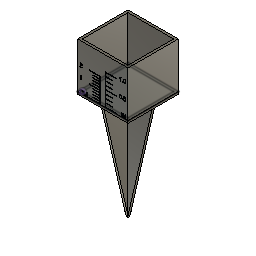
SprinklerGage (Autodesk Fusion 360 design; units mm, degrees)
Autodesk Fusion 360 part; units mm, degrees
sketch "Sketch1" plane through (0, 0, 0) normal (0, 0, 1) x (1, 0, 0)
  line L0 (0, 0) -> (38.1, 0)
  line L1 (38.1, 0) -> (38.1, 38.1)
  line L2 (38.1, 38.1) -> (0, 38.1)
  line L3 (0, 38.1) -> (0, 0)
  line L4 (-2, -2) -> (40.1, -2)
  line L5 (40.1, -2) -> (40.1, 40.1)
  line L6 (40.1, 40.1) -> (-2, 40.1)
  line L7 (-2, 40.1) -> (-2, -2)
  dimension "d6" = 38.1
  dimension "d7" = 38.1
  dimension "d8" = 2
  constraint horizontal L0
  constraint vertical L1
  constraint horizontal L2
  constraint vertical L3
  constraint coincident L0.start L3.end
  measures "d6" distance of L0.start L0.end
  measures "d7" distance of L0.start L2.end
extrude "Extrude1" add sketch "Sketch1" along normal blind 38.1 makes body 1
extrude "Extrude2" add sketch "Sketch1" against normal blind 2 contours L0 L1 L2 L3 | L4 L5 L6 L7 bodies 1
sketch "Sketch2" plane through (0, 0, -2) normal (0, 0, -1) x (1, 0, 0)
  line L0 (-2, 2) -> (-2, -40.1)
  line L1 (-2, -40.1) -> (40.1, -40.1)
  line L2 (40.1, -40.1) -> (40.1, 2)
  line L3 (40.1, 2) -> (-2, 2)
  line L4 (-2, 2) -> (18.05, 2)
  line L5 (18.05, 2) -> (18.05, -18.05)
  line L6 (18.05, -18.05) -> (-2, -18.05)
  line L7 (-2, -18.05) -> (-2, 2)
  line L8 (-2, -40.1) -> (18.05, -40.1)
  line L9 (18.05, -40.1) -> (18.05, -20.05)
  line L10 (18.05, -20.05) -> (-2, -20.05)
  line L11 (-2, -20.05) -> (-2, -40.1)
  line L12 (40.1, -40.1) -> (20.05, -40.1)
  line L13 (20.05, -40.1) -> (20.05, -20.05)
  line L14 (20.05, -20.05) -> (40.1, -20.05)
  line L15 (40.1, -20.05) -> (40.1, -40.1)
  line L16 (40.1, 2) -> (20.05, 2)
  line L17 (20.05, 2) -> (20.05, -18.05)
  line L18 (20.05, -18.05) -> (40.1, -18.05)
  line L19 (40.1, -18.05) -> (40.1, 2)
  dimension "d14" = 20.05
  dimension "d15" = 20.05
  dimension "d16" = 20.05
  dimension "d17" = 20.05
  dimension "d18" = 20.05
  dimension "d19" = 20.05
  dimension "d20" = 20.05
  dimension "d21" = 20.05
  constraint horizontal L4
  constraint vertical L5
  constraint horizontal L6
  constraint vertical L7
  constraint coincident L0.start L3.end
  constraint horizontal L8
  constraint vertical L9
  constraint horizontal L10
  constraint vertical L11
  constraint coincident L0.end L1.start
  constraint horizontal L12
  constraint vertical L13
  constraint horizontal L14
  constraint vertical L15
  constraint coincident L1.end L2.start
  constraint horizontal L16
  constraint vertical L17
  constraint horizontal L18
  constraint vertical L19
  constraint coincident L2.end L3.start
  measures "d14" distance of L0.start L4.end
  measures "d15" distance of L0.start L6.end
  measures "d16" distance of L0.end L8.end
  measures "d17" distance of L0.end L10.end
  measures "d18" distance of L1.end L12.end
  measures "d19" distance of L1.end L14.end
  measures "d20" distance of L2.end L16.end
  measures "d21" distance of L2.end L18.end
extrude "Extrude3" add sketch "Sketch2" along normal blind 88.9 separate body contours L0 L1 L2 L3 L5 L6 L9 L10 L13 L14 L17 L18 makes body 2
draft "Draft1" angle 13 neutral plane through (0, 0, -2) pull (0, 0, -1) 4 faces at (-2, 18.7167, -31.6333) (18.7167, 40.1, -31.6333) (40.1, 19.3833, -31.6333) (19.3833, -2, -31.6333) on bodies 2
sketch "Sketch3" plane through (0, -2, 0) normal (0, -1, 0) x (1, 0, 0)
  line L0 (40.1, -2) -> (40.1, 38.1)
  line L1 (40.1, 38.1) -> (-2, 38.1)
  line L2 (-2, 38.1) -> (-2, -2)
  line L3 (-2, -2) -> (40.1, -2)
  line L4 (-2, 0) -> (40.1, 0)
  line L5 (21.05, 0) -> (21.05, 25.4)
  line L6 (21.55, 0) -> (21.55, 25.4)
  line L7 (21.05, 0) -> (30.575, 0)
  line L8 (30.575, 0) -> (30.575, 0.5)
  line L9 (30.575, 0.5) -> (21.05, 0.5)
  line L10 (21.05, 0.5) -> (21.05, 0)
  line L11 (21.05, 25.4) -> (30.575, 25.4)
  line L12 (30.575, 25.4) -> (30.575, 25.9)
  line L13 (30.575, 25.9) -> (21.05, 25.9)
  line L14 (21.05, 25.9) -> (21.05, 25.4)
  line L15 (17.05, 0) -> (17.05, 20)
  line L16 (16.55, 0) -> (16.55, 20)
  line L17 (17.05, 0) -> (7.525, 0)
  line L18 (7.525, 0) -> (7.525, 0.5)
  line L19 (7.525, 0.5) -> (17.05, 0.5)
  line L20 (17.05, 0.5) -> (17.05, 0)
  line L21 (17.05, 20) -> (7.525, 20)
  line L22 (7.525, 20) -> (7.525, 20.5)
  line L23 (7.525, 20.5) -> (17.05, 20.5)
  line L24 (17.05, 20.5) -> (17.05, 20)
  line L25 (35.4718, 0) -> (38.195, 0) construction
  line L26 (38.195, 0) -> (38.195, 1.9986) construction
  line L27 (38.195, 1.9986) -> (35.4718, 1.9986) construction
  line L28 (35.4718, 1.9986) -> (35.4718, 0) construction
  line L29 (-0.095, 0) -> (3.87, 0) construction
  line L30 (3.87, 0) -> (3.87, 2) construction
  line L31 (3.87, 2) -> (-0.095, 2) construction
  line L32 (-0.095, 2) -> (-0.095, 0) construction
  line L33 (32.2448, 25.3469) -> (38.2256, 25.3396) construction
  line L34 (38.2256, 25.3396) -> (38.2281, 27.4199) construction
  line L35 (38.2281, 27.4199) -> (32.2474, 27.4272) construction
  line L36 (32.2474, 27.4272) -> (32.2448, 25.3469) construction
  line L37 (-0.095, 19.9302) -> (2.7186, 20.0383) construction
  line L38 (2.7186, 20.0383) -> (2.6413, 22.0491) construction
  line L39 (2.6413, 22.0491) -> (-0.1722, 21.9411) construction
  line L40 (-0.1722, 21.9411) -> (-0.095, 19.9302) construction
  line L41 (17.05, 10) -> (7.525, 10)
  line L42 (7.525, 10) -> (7.525, 10.5)
  line L43 (7.525, 10.5) -> (17.05, 10.5)
  line L44 (17.05, 10.5) -> (17.05, 10)
  line L45 (21.05, 12.7) -> (30.575, 12.7)
  line L46 (30.575, 12.7) -> (30.575, 13.2)
  line L47 (30.575, 13.2) -> (21.05, 13.2)
  line L48 (21.05, 13.2) -> (21.05, 12.7)
  line L49 (21.5697, 12.7) -> (38.195, 12.7) construction
  line L50 (38.195, 12.7) -> (38.195, 15.5) construction
  line L51 (38.195, 15.5) -> (21.5697, 15.5) construction
  line L52 (21.5697, 15.5) -> (21.5697, 12.7) construction
  line L53 (-0.095, 10) -> (3.9, 10) construction
  line L54 (3.9, 10) -> (3.9, 12.4) construction
  line L55 (3.9, 12.4) -> (-0.095, 12.4) construction
  line L56 (-0.095, 12.4) -> (-0.095, 10) construction
  line L57 (21.05, 6.35) -> (27.4, 6.35)
  line L58 (27.4, 6.35) -> (27.4, 6.85)
  line L59 (27.4, 6.85) -> (21.05, 6.85)
  line L60 (21.05, 6.85) -> (21.05, 6.35)
  line L61 (21.05, 9.525) -> (27.4, 9.525)
  line L62 (27.4, 9.525) -> (27.4, 10.025)
  line L63 (27.4, 10.025) -> (21.05, 10.025)
  line L64 (21.05, 10.025) -> (21.05, 9.525)
  line L65 (21.05, 3.175) -> (27.4, 3.175)
  line L66 (27.4, 3.175) -> (27.4, 3.675)
  line L67 (27.4, 3.675) -> (21.05, 3.675)
  line L68 (21.05, 3.675) -> (21.05, 3.175)
  line L69 (21.05, 15.875) -> (27.4, 15.875)
  line L70 (27.4, 15.875) -> (27.4, 16.375)
  line L71 (27.4, 16.375) -> (21.05, 16.375)
  line L72 (21.05, 16.375) -> (21.05, 15.875)
  line L73 (21.05, 19.05) -> (27.4, 19.05)
  line L74 (27.4, 19.05) -> (27.4, 19.55)
  line L75 (27.4, 19.55) -> (21.05, 19.55)
  line L76 (21.05, 19.55) -> (21.05, 19.05)
  line L77 (21.05, 22.225) -> (27.4, 22.225)
  line L78 (27.4, 22.225) -> (27.4, 22.725)
  line L79 (27.4, 22.725) -> (21.05, 22.725)
  line L80 (21.05, 22.725) -> (21.05, 22.225)
  line L81 (17.05, 2) -> (10.7, 2)
  line L82 (10.7, 2) -> (10.7, 2.5)
  line L83 (10.7, 2.5) -> (17.05, 2.5)
  line L84 (17.05, 2.5) -> (17.05, 2)
  line L85 (17.05, 4) -> (10.7, 4)
  line L86 (10.7, 4) -> (10.7, 4.5)
  line L87 (10.7, 4.5) -> (17.05, 4.5)
  line L88 (17.05, 4.5) -> (17.05, 4)
  line L89 (17.05, 6) -> (10.7, 6)
  line L90 (10.7, 6) -> (10.7, 6.5)
  line L91 (10.7, 6.5) -> (17.05, 6.5)
  line L92 (17.05, 6.5) -> (17.05, 6)
  line L93 (17.05, 8) -> (10.7, 8)
  line L94 (10.7, 8) -> (10.7, 8.5)
  line L95 (10.7, 8.5) -> (17.05, 8.5)
  line L96 (17.05, 8.5) -> (17.05, 8)
  line L97 (17.05, 12) -> (10.7, 12)
  line L98 (10.7, 12) -> (10.7, 12.5)
  line L99 (10.7, 12.5) -> (17.05, 12.5)
  line L100 (17.05, 12.5) -> (17.05, 12)
  line L101 (17.05, 14) -> (10.7, 14)
  line L102 (10.7, 14) -> (10.7, 14.5)
  line L103 (10.7, 14.5) -> (17.05, 14.5)
  line L104 (17.05, 14.5) -> (17.05, 14)
  line L105 (17.05, 16) -> (10.7, 16)
  line L106 (10.7, 16) -> (10.7, 16.5)
  line L107 (10.7, 16.5) -> (17.05, 16.5)
  line L108 (17.05, 16.5) -> (17.05, 16)
  line L109 (17.05, 18) -> (10.7, 18)
  line L110 (10.7, 18) -> (10.7, 18.5)
  line L111 (10.7, 18.5) -> (17.05, 18.5)
  line L112 (17.05, 18.5) -> (17.05, 18)
  point P0 (17.05, 0)
  point P1 (-2, 0)
  point P2 (21.05, 0)
  point P3 (40.1, 0)
  point P4 (17.05, 10)
  point P5 (21.05, 12.7)
  point P6 (21.05, 0)
  point P7 (21.05, 0.25)
  point P8 (21.05, 6.35)
  point P9 (21.05, 9.525)
  point P10 (21.05, 19.05)
  point P11 (21.05, 15.875)
  point P12 (21.05, 3.175)
  point P13 (21.05, 22.225)
  point P14 (17.05, 2)
  point P15 (17.05, 4)
  point P16 (17.05, 6)
  point P17 (17.05, 8)
  point P18 (17.05, 9.1)
  point P19 (17.05, 18)
  point P20 (17.05, 16)
  point P21 (17.05, 14)
  point P22 (17.05, 12)
  dimension "d27" = 19.05
  dimension "d29" = 19.05
  dimension "d30" = 25.4
  dimension "d31" = 0.5
  dimension "d32" = 9.525
  dimension "d33" = 0.5
  dimension "d34" = 9.525
  dimension "d35" = 0.5
  dimension "d37" = 20
  dimension "d39" = 9.525
  dimension "d40" = 0.5
  dimension "d41" = 9.525
  dimension "d42" = 0.5
  dimension "d45" = 3
  dimension "d46" = 1.905
  dimension "d47" = 3
  dimension "d48" = 1.905
  dimension "d49" = 3
  dimension "d50" = 0.069
  dimension "d51" = 1.905
  dimension "d52" = 3
  dimension "d53" = 10
  dimension "d54" = 9.525
  dimension "d55" = 0.5
  dimension "d56" = 12.7
  dimension "d57" = 0.25
  dimension "d58" = 9.525
  dimension "d59" = 0.5
  dimension "d60" = 3
  dimension "d61" = 1.905
  dimension "d62" = 3
  dimension "d63" = 1.905
  dimension "d65" = 1.905
  dimension "d66" = 6.35
  dimension "d67" = 0.5
  dimension "d68" = 3.175
  dimension "d69" = 6.35
  dimension "d70" = 9.525
  dimension "d71" = 6.35
  dimension "d72" = 0.5
  dimension "d73" = 6.35
  dimension "d74" = 0.5
  dimension "d75" = 3.175
  dimension "d76" = 6.35
  dimension "d77" = 9.525
  dimension "d78" = 6.35
  dimension "d79" = 0.5
  dimension "d80" = 6.35
  dimension "d81" = 0.5
  dimension "d82" = 6.35
  dimension "d83" = 0.5
  dimension "d84" = 2
  dimension "d85" = 4
  dimension "d86" = 6
  dimension "d87" = 8
  dimension "d88" = 6.35
  dimension "d89" = 0.5
  dimension "d90" = 6.35
  dimension "d91" = 0.5
  dimension "d92" = 6.35
  dimension "d93" = 0.5
  dimension "d94" = 6.35
  dimension "d95" = 0.5
  dimension "d96" = 2
  dimension "d97" = 4
  dimension "d98" = 6
  dimension "d99" = 8
  dimension "d100" = 6.35
  dimension "d101" = 0.5
  dimension "d102" = 6.35
  dimension "d103" = 0.5
  dimension "d104" = 6.35
  dimension "d105" = 0.5
  dimension "d106" = 6.35
  dimension "d107" = 0.5
  text T0 "IN" font "Arial" height 3 align right bottom in box 2.7232 x 1.9986 at (35.4718, 0) x (1, 0) y (0, 1) spacing 1 kerned
  text T1 "CM." font "Arial" height 3 align left bottom in box 3.965 x 2 at (-0.095, 0) x (1, 0) y (0, 1) spacing 1 kerned
  text T2 "1.0" font "Arial" height 3 align right bottom in box 5.9808 x 2.0803 at (32.2448, 25.3469) x (0.999999, -0.001209) y (0.001209, 0.999999) spacing 1 kerned
  text T3 "2" font "Arial" height 3 align left top in box 2.8156 x 2.0123 at (-0.095, 19.9302) x (0.999264, 0.038371) y (-0.038371, 0.999264) spacing 1 kerned
  text T4 "0.5" font "Arial" height 3 align right bottom in box 16.6253 x 2.8 at (21.5697, 12.7) x (1, 0) y (0, 1) spacing 1 kerned
  text T5 "1" font "Arial" height 3 align left bottom in box 3.995 x 2.4 at (-0.095, 10) x (1, 0) y (0, 1) spacing 1 kerned
  constraint coincident P0 L4
  constraint coincident L4 P6
  constraint coincident P6 P2
  constraint perpendicular L4 L5
  constraint horizontal L7
  constraint vertical L8
  constraint horizontal L9
  constraint vertical L10
  constraint horizontal L11
  constraint vertical L12
  constraint horizontal L13
  constraint vertical L14
  constraint coincident P0 L15.start
  constraint perpendicular L4 L15
  constraint horizontal L17
  constraint vertical L18
  constraint horizontal L19
  constraint vertical L20
  constraint horizontal L21
  constraint vertical L22
  constraint horizontal L23
  constraint vertical L24
  constraint coincident L4
  constraint coincident L15 P4
  constraint horizontal L41
  constraint vertical L42
  constraint horizontal L43
  constraint vertical L44
  constraint coincident P4 L41.start
  constraint coincident L5 P5
  constraint coincident L5 P7
  constraint horizontal L45
  constraint vertical L46
  constraint horizontal L47
  constraint vertical L48
  constraint coincident P5 L45.start
  constraint coincident L5 P8
  constraint coincident L5 P9
  constraint coincident L5 P10
  constraint coincident L5 P11
  constraint coincident L5 P12
  constraint horizontal L57
  constraint vertical L58
  constraint horizontal L59
  constraint vertical L60
  constraint coincident P8 L57.start
  constraint horizontal L61
  constraint vertical L62
  constraint horizontal L63
  constraint vertical L64
  constraint coincident P9 L61.start
  constraint horizontal L65
  constraint vertical L66
  constraint horizontal L67
  constraint vertical L68
  constraint coincident P12 L65.start
  constraint coincident L5 P13
  constraint horizontal L69
  constraint vertical L70
  constraint horizontal L71
  constraint vertical L72
  constraint coincident P11 L69.start
  constraint horizontal L73
  constraint vertical L74
  constraint horizontal L75
  constraint vertical L76
  constraint coincident P10 L73.start
  constraint horizontal L77
  constraint vertical L78
  constraint horizontal L79
  constraint vertical L80
  constraint coincident P13 L77.start
  constraint coincident L15 P14
  constraint coincident L15 P15
  constraint coincident L15 P16
  constraint coincident L15 P17
  constraint coincident L15 P18
  constraint horizontal L81
  constraint vertical L82
  constraint horizontal L83
  constraint vertical L84
  constraint coincident P14 L81.start
  constraint horizontal L85
  constraint vertical L86
  constraint horizontal L87
  constraint vertical L88
  constraint coincident P15 L85.start
  constraint horizontal L89
  constraint vertical L90
  constraint horizontal L91
  constraint vertical L92
  constraint coincident P16 L89.start
  constraint horizontal L93
  constraint vertical L94
  constraint horizontal L95
  constraint vertical L96
  constraint coincident P17 L93.start
  constraint coincident L15 P19
  constraint coincident L15 P20
  constraint coincident L15 P21
  constraint coincident L15 P22
  constraint horizontal L97
  constraint vertical L98
  constraint horizontal L99
  constraint vertical L100
  constraint coincident P22 L97.start
  constraint horizontal L101
  constraint vertical L102
  constraint horizontal L103
  constraint vertical L104
  constraint coincident P21 L101.start
  constraint horizontal L105
  constraint vertical L106
  constraint horizontal L107
  constraint vertical L108
  constraint coincident P20 L105.start
  constraint horizontal L109
  constraint vertical L110
  constraint horizontal L111
  constraint vertical L112
  constraint coincident P19 L109.start
  measures "d27" distance of P0 P1
  measures "d29" distance of P6 P3
  measures "d30" distance of P6 L5.end
  measures "d32" distance of P6 L7.end
  measures "d33" distance of P6 L9.end
  measures "d34" distance of L5.end L11.end
  measures "d35" distance of L5.end L13.end
  measures "d37" distance of P0 L15.end
  measures "d39" distance of P0 L17.end
  measures "d40" distance of P0 L19.end
  measures "d41" distance of L15.end L21.end
  measures "d42" distance of L15.end L23.end
  measures "d46" distance of P3 L26
  measures "d48" distance of L2 L32
  measures "d50" angle of L0 L34
  measures "d51" distance of P3 L34
  measures "d53" distance of P0 P4
  measures "d54" distance of P4 L41.end
  measures "d55" distance of P4 L43.end
  measures "d56" distance of P6 P5
  measures "d57" distance of P6 P7
  measures "d58" distance of P5 L45.end
  measures "d59" distance of P5 L47.end
  measures "d61" distance of L0 L50
  measures "d63" distance of L2 L56
  measures "d66" distance of P8 L57.end
  measures "d67" distance of P8 L59.end
  measures "d68" distance of P6 P12
  measures "d69" distance of P6 P8
  measures "d70" distance of P6 P9
  measures "d71" distance of P9 L61.end
  measures "d72" distance of P9 L63.end
  measures "d73" distance of P12 L65.end
  measures "d74" distance of P12 L67.end
  measures "d75" distance of P5 P11
  measures "d76" distance of P5 P10
  measures "d77" distance of P5 P13
  measures "d78" distance of P11 L69.end
  measures "d79" distance of P11 L71.end
  measures "d80" distance of P10 L73.end
  measures "d81" distance of P10 L75.end
  measures "d82" distance of P13 L77.end
  measures "d83" distance of P13 L79.end
  measures "d84" distance of P0 P14
  measures "d85" distance of P0 P15
  measures "d86" distance of P0 P16
  measures "d87" distance of P0 P17
  measures "d88" distance of P14 L81.end
  measures "d89" distance of P14 L83.end
  measures "d90" distance of P15 L85.end
  measures "d91" distance of P15 L87.end
  measures "d92" distance of P16 L89.end
  measures "d93" distance of P16 L91.end
  measures "d94" distance of P17 L93.end
  measures "d95" distance of P17 L95.end
  measures "d96" distance of P4 P22
  measures "d97" distance of P4 P21
  measures "d98" distance of P4 P20
  measures "d99" distance of P4 P19
  measures "d100" distance of P22 L97.end
  measures "d101" distance of P22 L99.end
  measures "d102" distance of P21 L101.end
  measures "d103" distance of P21 L103.end
  measures "d104" distance of P20 L105.end
  measures "d105" distance of P20 L107.end
  measures "d106" distance of P19 L109.end
  measures "d107" distance of P19 L111.end
extrude "Extrude4" cut sketch "Sketch3" sketch "Sketch3" against normal blind 1 contours L4 L6 L7 L8 L9 | L4 L5 L6 L7 L9 L10 | L4 L16 L17 L18 L19 | L5 L6 L9 L65 | L4 L15 L16 L17 L19 L20 | L5 L6 L65 L67 L68 | L6 L65 L66 L67 | L15 L16 L19 L81 | L5 L6 L57 L67 | L16 L81 L82 L83 | L15 L16 L81 L83 L84 | L5 L6 L57 L59 L60 | L6 L57 L58 L59 | L15 L16 L83 L85 | L5 L6 L59 L61 | L16 L85 L86 L87 | L15 L16 L85 L87 L88 | L5 L6 L61 L63 L64 | L6 L61 L62 L63 | L15 L16 L87 L89 | L5 L6 L45 L63 | L16 L89 L90 L91 | L15 L16 L89 L91 L92 | L5 L6 L45 L47 L48 | L6 L45 L46 L47 | L15 L16 L91 L93 | L5 L6 L47 L69 | L16 L93 L94 L95 | L15 L16 L93 L95 L96 | L5 L6 L69 L71 L72 | L6 L69 L70 L71 | L15 L16 L41 L95 | L5 L6 L71 L73 | L16 L41 L42 L43 | L15 L16 L41 L43 L44 | L5 L6 L73 L75 L76 | L6 L73 L74 L75 | L15 L16 L43 L97 | L5 L6 L75 L77 | L16 L97 L98 L99 | L15 L16 L97 L99 L100 | L5 L6 L77 L79 L80 | L6 L77 L78 L79 | L15 L16 L99 L101 | L5 L6 L11 L79 | L16 L101 L102 L103 | L15 L16 L101 L103 L104 | L11 L12 L13 L14 | L15 L16 L103 L105 | L16 L105 L106 L107 | L15 L16 L105 L107 L108 | L15 L16 L107 L109 | L16 L109 L110 L111 | L15 L16 L109 L111 L112 | L15 L16 L21 L111 | L21 L22 L23 L24 of sketch 2 text T1 T0 T3 T2 T4 T5 bodies 1
equation "length = 1.5 in"
equation "width = 1.5 in"
equation "height = 1.5 in"
equation "thickness = 2 mm"
equation "spike_length = 3.5 in"
equation "d6 = width"
equation "d7 = length"
equation "d8 = thickness"
equation "d9 = height"
equation "d11 = -thickness"
equation "Spike_top = ( width + thickness ) / 2"
equation "d14 = Spike_top"
equation "d15 = Spike_top"
equation "d16 = Spike_top"
equation "d17 = Spike_top"
equation "d18 = Spike_top"
equation "d19 = Spike_top"
equation "d20 = Spike_top"
equation "d21 = Spike_top"
equation "d22 = spike_length"
equation "d24 = spike_draft"
equation "spike_draft = 13 deg"
equation "d27 = ( width / 2 )"
equation "line_thickness = 0.5 mm"
equation "d29 = width / 2"
equation "d31 = line_thickness"
equation "d32 = width / 4"
equation "d33 = line_thickness"
equation "d34 = width / 4"
equation "d35 = line_thickness"
equation "emboss = 1 mm"
equation "d38 = -line_thickness"
equation "d39 = width / 4"
equation "d40 = line_thickness"
equation "d41 = width / 4"
equation "d42 = line_thickness"
equation "d43 = -emboss"
equation "d45 = text_height"
equation "d46 = width / 20"
equation "d47 = text_height"
equation "d48 = width / 20"
equation "d49 = text_height"
equation "d51 = width / 20"
equation "d52 = text_height"
equation "d54 = width / 4"
equation "d55 = line_thickness"
equation "d57 = ( 0.5 / 2 ) * 1 mm"
equation "d58 = width / 4"
equation "d59 = line_thickness"
equation "d60 = text_height"
equation "d61 = width / 20"
equation "d62 = text_height"
equation "d63 = width / 20"
equation "d65 = width / 20"
equation "d66 = width / 6"
equation "d67 = line_thickness"
equation "d68 = 0.5 in / 4"
equation "d69 = 0.5 in / 2"
equation "d70 = 0.5 in * 0.75"
equation "d71 = width / 6"
equation "d72 = line_thickness"
equation "d73 = width / 6"
equation "d74 = line_thickness"
equation "d75 = 0.5 in * 0.25"
equation "d76 = 0.5 in * 0.5"
equation "d77 = 0.5 in * 0.75"
equation "d78 = width / 6"
equation "d79 = line_thickness"
equation "d80 = width / 6"
equation "d81 = line_thickness"
equation "d82 = width / 6"
equation "d83 = line_thickness"
equation "d88 = width / 6"
equation "d89 = line_thickness"
equation "d90 = width / 6"
equation "d91 = line_thickness"
equation "d92 = width / 6"
equation "d93 = line_thickness"
equation "d94 = width / 6"
equation "d95 = line_thickness"
equation "d100 = width / 6"
equation "d101 = line_thickness"
equation "d102 = width / 6"
equation "d103 = line_thickness"
equation "d104 = width / 6"
equation "d105 = line_thickness"
equation "d106 = width / 6"
equation "d107 = line_thickness"
equation "text_height = 3 mm"
